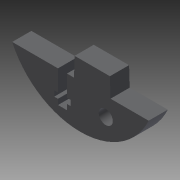
# Autodesk Inventor part: trzymacz_bowdena
Saved by Autodesk Inventor 2013 (Build 170138000, 138)
## iProperties
Created: 2013-09-02
Part Number: trzymacz_bowdena
Material: Generic
Document SubType Name: Modeling
Designer: dzban
Density: 1 g/cm^3
Author: dzban
Autodesk Inventor part; units mm, degrees
ref_plane "YZ Plane" through (0, 0, 0) normal (1, 0, 0) x (0, 1, 0)
ref_plane "XZ Plane" through (0, 0, 0) normal (0, 1, 0) x (-1, 0, 0)
ref_plane "XY Plane" through (0, 0, 0) normal (0, 0, 1) x (1, 0, 0)
sketch "Sketch1" plane through (0, 0, 0) normal (0, 1, 0) x (-1, 0, 0)
  line L0 (0, 0) -> (2.35, 0)
  line L1 (2.35, 0) -> (2.65, 6.4)
  line L2 (2.65, 6.4) -> (14.45, 6.4)
  line L3 (14.45, 6.4) -> (14.75, 0)
  line L4 (14.75, 0) -> (17, 0)
  line L5 (17, 0) -> (17, -7)
  line L6 (17, -7) -> (15.75, -7)
  line L7 (15.75, -7) -> (15.75, -8.8)
  line L8 (15.75, -8.8) -> (17, -8.8)
  line L9 (17, -8.8) -> (17, -10.6)
  line L10 (17, -10.6) -> (20, -10.6)
  line L11 (20, -10.6) -> (20, -8.8)
  line L12 (20, -8.8) -> (21.25, -8.8)
  line L13 (21.25, -8.8) -> (21.25, -7)
  line L14 (21.25, -7) -> (20, -7)
  line L15 (20, -7) -> (20, 0)
  line L16 (20, 0) -> (25, 0)
  line L17 (25, 0) -> (25, -15)
  line L18 (25, -15) -> (0, -15)
  line L19 (0, -15) -> (0, 0)
  circle A0 centre (4.0344, -6.0871) radius 2.35
  dimension "d0" = 7
  dimension "d2" = 1.8
  dimension "d3" = 1.8
  dimension "d4" = 3
  dimension "d5" = 1.25
  dimension "d6" = 1.25
  dimension "d7" = 25
  dimension "d8" = 15
  dimension "d9" = 5
  dimension "d10" = 11.8
  dimension "d11" = 12.4
  dimension "d12" = 6.4
  dimension "d14" = 2.25
  dimension "d15" = 4.7
  dimension "d26" = 2.35
  constraints: 40 end point, 11 perpendicular, 5 collinear, 2 horizontal, 1 centre point
  measures "d0" distance between parallel lines of L16 L14
  measures "d2" distance between parallel lines of L12 L14
  measures "d3" distance between parallel lines of L12 L10
  measures "d4" distance between parallel lines of L15 L5
  measures "d5" distance between parallel lines of L11 L13
  measures "d6" distance between parallel lines of L7 L9
  measures "d7" distance between parallel lines of L17 L19
  measures "d8" distance between parallel lines of L18 L0
  measures "d9" distance between parallel lines of L17 L15
  measures "d10" distance of L2.end L1.end
  measures "d11" distance of L3.end L0.end
  measures "d12" distance between parallel lines of L2 L0
  measures "d14" distance from line of L3.end L5
  measures "d15" diameter of A0
  measures "d26" distance from line of L19 L0.end
extrude "Extrusion1" add sketch "Sketch1" along normal blind 6.4
fillet "Fillet1" radius 2 2 edges at (-25, 3.2, -15) (0, 3.2, -15)
sketch "Sketch2" plane through (0, 6.4, 0) normal (0, 1, 0) x (1, 0, 0)
  line L0 (-25, 13) -> (-25, 0) projected
  line L1 (0, 0) -> (0, 13) projected
  circle A0 centre (-12.5, -10.4574) radius 25.0744
  line L2 (-25, 0) -> (-35.2897, 0)
  line L3 (-25, 0) -> (-25, 11.2791)
  line L4 (0, 0) -> (0, 11.2791)
  line L5 (0, 0) -> (10.2897, 0)
  dimension "d19" = 12.5
  constraints: 8 end point, 4 point on circle, 2 perpendicular, 2 point on line, 1 centre point
  measures "d19" distance from line of L4 A0.centre
extrude "Extrusion2" add sketch "Sketch2" against normal blind 6.4 contours L0 L2 A0 | A0 L5 L1
sketch "Sketch3" plane through (0, 6.4, 0) normal (0, 1, 0) x (1, 0, 0)
  arc A0 (0, 13) -> (-2, 15) centre (-2, 13) ccw projected
  line L0 (-2, 15) -> (-23, 15) projected
  arc A1 (-23, 15) -> (-25, 13) centre (-23, 13) ccw projected
  line L1 (-25, 13) -> (-25, 11.2791) projected
  line L2 (0, 11.2791) -> (0, 13) projected
  circle A2 centre (-12.5, -10.4574) radius 25.0744 projected
  point P0 (0, 0)
extrude "Extrusion3" cut sketch "Sketch3" against normal blind 6.4 contours L2 A2 L1 A1 L0 A0
sketch "Sketch4" plane through (0, 0, 0) normal (0, -1, 0) x (1, 0, 0)
  line L0 (10.2897, 0) -> (-2.35, 0) projected
  line L1 (-2.35, 0) -> (-2.65, 6.4) projected
  line L2 (-14.45, 6.4) -> (-14.75, 0) projected
  line L3 (-14.75, 0) -> (-17, 0) projected
  line L4 (-14.45, 6.4) -> (-14.65, 0)
  line L5 (-14.65, 0) -> (-14.75, 0)
  line L6 (-2.65, 6.4) -> (-2.45, 0)
  line L7 (-2.45, 0) -> (-2.35, 0)
  point P0 (0, 0)
  dimension "d27" = 0.1
  dimension "d28" = 0.1
  constraints: 8 end point, 2 collinear
  measures "d27" distance of L4.end L2.end
  measures "d28" distance of L0.end L6.end
extrude "Extrusion4" cut sketch "Sketch4" against normal blind 10
body "Solid1"
